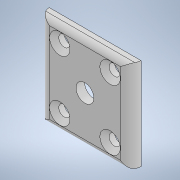
# Autodesk Inventor part: Крышка поворотного кулака
Saved by Autodesk Inventor 2020 (Build 240168000, 168)
## iProperties
Created: 2021-04-25
Part Number: Крышка поворотного кулака
Material: Типовые
Document SubType Name: Modeling
Designer: Антон
Density: 1 g/cm^3
Appearance: По умолчанию
Author: Антон
Autodesk Inventor part; units mm, degrees
ref_plane "YZ Plane" through (0, 0, 0) normal (1, 0, 0) x (0, 1, 0)
ref_plane "XZ Plane" through (0, 0, 0) normal (0, 1, 0) x (-1, 0, 0)
ref_plane "XY Plane" through (0, 0, 0) normal (0, 0, 1) x (1, 0, 0)
sketch "Эскиз1" plane through (0, 0, 0) normal (0, 0, 1) x (1, 0, 0)
  line L0 (0, 0) -> (18, 0)
  line L1 (18, 0) -> (18, 18)
  line L2 (18, 18) -> (0, 18)
  line L3 (0, 18) -> (0, 0)
  dimension "d0" = 18
  dimension "d1" = 18
  constraints: 8 end point, 2 parallel, 1 horizontal, 1 perpendicular
  measures "d0" distance of L2.end L1.end
  measures "d1" distance of L1.end L0.end
extrude "Выдавливание1" add sketch "Эскиз1" along normal blind 2
sketch "Эскиз4" plane through (0, 0, 0) normal (0, 0, -1) x (-1, 0, 0)
  circle A0 centre (-9, 9) radius 4.05
  line L0 (-18, 0) -> (-18, 18) projected
  line L1 (-18, 9) -> (0, 9)
  line L2 (0, 18) -> (0, 0) projected
  dimension "d14" = 8.1
  constraints: 3 midpoint, 2 end point, 1 centre point, 1 coincident
  measures "d14" diameter of A0
extrude "Выдавливание3" cut sketch "Эскиз4" against normal blind 0.3
sketch "Эскиз5" plane through (0, 0, 2) normal (0, 0, 1) x (1, 0, 0)
  circle A0 centre (9, 9) radius 1.75 projected
  circle A1 centre (9, 9) radius 5.714 projected
  line L0 (0, 18) -> (0, 0) projected
  line L1 (6.1362, 11.8638) -> (0, 18)
  line L2 (18, 0) -> (18, 18) projected
  line L3 (11.8638, 11.8638) -> (18, 18)
  line L4 (0, 0) -> (18, 0) projected
  line L5 (0, 0) -> (6.1362, 6.1362)
  line L6 (18, 0) -> (11.8638, 6.1362)
  circle A2 centre (9, 9) radius 4.05 projected
  line L7 (3.0681, 14.9319) -> (4.0681, 14.9319)
  line L8 (3.0681, 3.0681) -> (4.0681, 3.0681)
  line L9 (14.9319, 3.0681) -> (13.9319, 3.0681)
  line L10 (14.9319, 14.9319) -> (13.9319, 14.9319)
  dimension "d24" = 1
  constraints: 16 end point, 4 horizontal, 4 midpoint, 4 point on circle, 3 equal length, 2 collinear
  measures "d24" distance of L7.start L7.end
hole "Отверстие2" at (4.0681, 14.9319, 2) at (4.0681, 3.0681, 2) at (13.9319, 14.9319, 2) at (13.9319, 3.0681, 2) direction (0, 0, -1) diameter 2.2 depth 5 countersink diameter 4 countersink angle 90
fillet "Сопряжение1" radius 1.05 2 edges at (9, 0, 2) (9, 18, 2)
fillet "Сопряжение1" radius 2.05 2 edges at (18, 9, 2) (0, 9, 2)
sketch "Эскиз6" plane through (9, 9, 0.3) normal (0, 0, -1) x (-1, 0, 0)
  circle A0 centre (0, 0) radius 1.75
  point P0 (9, -9)
  dimension "d27" = 3.5
  constraints: 1 centre point
  measures "d27" diameter of A0
extrude "Выдавливание4" cut sketch "Эскиз6" against normal through all
